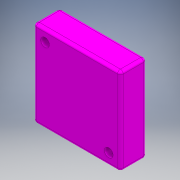
# Autodesk Inventor part: calle-patin
Saved by Autodesk Inventor 2019 (Build 230136000, 136)
## iProperties
Created: 2018-04-14
Part Number: calle-patin
Material: Générique
Document SubType Name: Modeling
Designer: franc
Density: 1 g/cm^3
Appearance: Par défaut
Author: franc
Autodesk Inventor part; units mm, degrees
ref_plane "YZ Plane" through (0, 0, 0) normal (1, 0, 0) x (0, 1, 0)
ref_plane "XZ Plane" through (0, 0, 0) normal (0, 1, 0) x (-1, 0, 0)
ref_plane "XY Plane" through (0, 0, 0) normal (0, 0, 1) x (1, 0, 0)
sketch "Esquisse1" plane through (0, 0, 0) normal (0, 1, 0) x (-1, 0, 0)
  line L0 (7.7669, 18.1799) -> (-22.2331, 18.1799)
  line L1 (-22.2331, 18.1799) -> (-22.2331, -11.8201)
  line L2 (-22.2331, -11.8201) -> (7.7669, -11.8201)
  line L3 (7.7669, -11.8201) -> (7.7669, 18.1799)
  point P0 (0, 0)
  dimension "d0" = 30
  dimension "d1" = 30
  constraints: 8 end point, 2 parallel, 1 horizontal, 1 perpendicular
  measures "d0" distance of L2.end L1.end
  measures "d1" distance of L2.end L0.start
extrude "Extrusion1" add sketch "Esquisse1" along normal blind 9
sketch "Esquisse2" plane through (0, 9, 0) normal (0, 1, 0) x (1, 0, 0)
  circle A0 centre (-3.7669, -14.1799) radius 1.5
  circle A1 centre (18.2331, 7.8201) radius 1.5
  line L0 (-7.7669, 11.8201) -> (-7.7669, -18.1799) projected
  line L1 (-7.7669, -18.1799) -> (22.2331, -18.1799) projected
  line L2 (22.2331, 11.8201) -> (-7.7669, 11.8201) projected
  line L3 (22.2331, -18.1799) -> (22.2331, 11.8201) projected
  point P0 (0, 0)
  dimension "d4" = 3
  dimension "d5" = 3
  dimension "d6" = 4
  dimension "d8" = 4
  dimension "d9" = 4
  dimension "d13" = 4
  constraints: 2 centre point
  measures "d4" diameter of A0
  measures "d5" diameter of A1
  measures "d6" distance from line of L0 A0.centre
  measures "d8" distance from line of L1 A0.centre
  measures "d9" distance from line of L2 A1.centre
  measures "d13" distance from line of L3 A1.centre
extrude "Extrusion2" cut sketch "Esquisse2" against normal blind 10 contours A0 | A1
fillet "Congé1" radius 1 12 edges at (7.2331, 9, 18.1799) (22.2331, 9, 3.1799) (7.2331, 9, -11.8201) (-7.7669, 9, 3.1799) (-7.7669, 0, 3.1799) (7.2331, 0, -11.8201) (22.2331, 0, 3.1799) (7.2331, 0, 18.1799) (22.2331, 4.5, 18.1799) (22.2331, 4.5, -11.8201) (-7.7669, 4.5, -11.8201) (-7.7669, 4.5, 18.1799)
